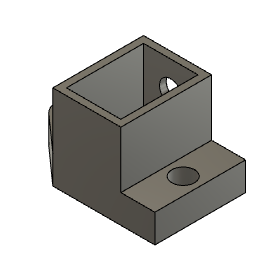
drawing_28 (Autodesk Fusion 360 design; units mm, degrees)
Autodesk Fusion 360 part; units mm, degrees
sketch "Sketch1" plane through (0, 0, 0) normal (0, 1, 0) x (1, 0, 0)
  line L0 (-15, -40) -> (60, -40)
  line L1 (60, -40) -> (60, 40)
  line L2 (60, 40) -> (-15, 40)
  line L3 (-60, -40) -> (60, 40) construction
  line L4 (60, -40) -> (-60, 40) construction
  line L5 (-60, 0) -> (-45, 0) construction
  line L6 (-45, 0) -> (-45, 13.3333) construction
  line L7 (-15, -40) -> (-15, 40)
  line L8 (-47.3875, 11.2111) -> (-15, 40)
  line L9 (-47.3875, -11.2111) -> (-15, -40)
  arc A0 (-47.3875, 11.2111) -> (-47.3875, -11.2111) centre (-37.422, 0) ccw
  circle A1 centre (-37.422, 0) radius 10
  dimension "d1" = 120
  dimension "d2" = 80
  dimension "d3" = 15
  dimension "d4" = 20
  constraint horizontal L0
  constraint perpendicular L0 L1
  constraint parallel L0 L2
  constraint coincident L3 origin
  constraint coincident L4 origin
  constraint perpendicular L2 L6
  constraint coincident L8 L6.end
  constraint coincident L5.start L8
  constraint coincident L5.start L9
  constraint tangent L8 A0
  constraint tangent L9 A0
  constraint concentric A0 A1
  measures "d1" distance of L1.end L4.end
  measures "d2" distance of L0.end L1.end
  measures "d3" radius of A0
  measures "d4" diameter of A1
extrude "Extrude1" add sketch "Sketch1" along normal blind 25
extrude "Extrude2" add 1 faces at (60, 8.3333, 13.3333) along direction (1, 0, 0) blind 15
sketch "Sketch3" plane through (0, 25, 0) normal (0, 1, 0) x (-1, 0, 0)
  circle A0 centre (37.422, 0) radius 10
  arc A1 (47.3875, -11.2111) -> (47.3875, 11.2111) centre (37.422, 0) ccw
  line L0 (47.3875, 11.2111) -> (15, 40)
  line L1 (15, 40) -> (-75, 40)
  line L2 (-75, 40) -> (-75, -40)
  line L3 (-75, -40) -> (15, -40)
  line L4 (15, -40) -> (47.3875, -11.2111)
  line L5 (-75, 0) -> (-60, 0) construction
  circle A2 centre (-60, 0) radius 10
  dimension "d10" = 15
  dimension "d11" = 20
  constraint midpoint L2 L5.start
  constraint perpendicular L2 L5
  constraint coincident L5.end A2.centre
  measures "d10" distance of L5.start L5.end
  measures "d11" diameter of A2
extrude "Extrude3" cut sketch "Sketch3" against normal blind 55 contours A2
sketch "Sketch4" plane through (0, 25, 0) normal (0, 1, 0) x (-1, 0, 0)
  circle A0 centre (-60, 0) radius 10
  circle A1 centre (37.422, 0) radius 10
  arc A2 (47.3875, -11.2111) -> (47.3875, 11.2111) centre (37.422, 0) ccw
  line L0 (47.3875, 11.2111) -> (15, 40)
  line L1 (15, 40) -> (-75, 40)
  line L2 (-75, 40) -> (-75, -40)
  line L3 (-75, -40) -> (15, -40)
  line L4 (15, -40) -> (47.3875, -11.2111)
  line L5 (15, 40) -> (-45, 40)
  line L6 (-45, 40) -> (-45, -40)
  line L7 (-45, -40) -> (15, -40)
  line L8 (15, -40) -> (15, 40)
  line L9 (15, 40) -> (-45, -40) construction
  line L10 (-45, 40) -> (15, -40) construction
  point P0 (-15, 0)
  constraint horizontal L5
  constraint perpendicular L5 L6
  constraint parallel L5 L7
  constraint parallel L6 L8
  constraint coincident L0.end L1.start
  constraint coincident L9 P0
  constraint coincident L10 P0
extrude "Extrude4" add sketch "Sketch4" along normal blind 50 contours L1 L3 L5 L6 L7 L8
shell "Shell1" thickness 6 removed faces 1 at (5, 75, -13.3333)
sketch "Sketch5" plane through (0, 6, 0) normal (0, 1, 0) x (-1, 0, 0)
  line L0 (33.514, 15.5154) -> (12.7188, 34)
  line L1 (12.7188, 34) -> (-69, 34)
  line L2 (-69, 34) -> (-69, 13.2288)
  arc A0 (-69, -13.2288) -> (-69, 13.2288) centre (-60, 0) ccw
  line L3 (-69, -13.2288) -> (-69, -34)
  line L4 (-69, -34) -> (12.7188, -34)
  line L5 (12.7188, -34) -> (33.514, -15.5154)
  arc A1 (33.514, 15.5154) -> (33.514, -15.5154) centre (37.422, 0) ccw
  line L6 (-15, -40) -> (-15, -16) construction
  line L7 (-2.5, -3.5) -> (-27.5, -3.5)
  line L8 (-27.5, -3.5) -> (-27.5, -28.5)
  line L9 (-27.5, -28.5) -> (-2.5, -28.5)
  line L10 (-2.5, -28.5) -> (-2.5, -3.5)
  line L11 (-2.5, -3.5) -> (-27.5, -28.5) construction
  line L12 (-27.5, -3.5) -> (-2.5, -28.5) construction
  point P0 (-15, -16)
  dimension "d17" = 24
  dimension "d18" = 25
  dimension "d19" = 25
  constraint perpendicular L4 L6
  constraint horizontal L7
  constraint perpendicular L7 L8
  constraint parallel L7 L9
  constraint parallel L8 L10
  constraint coincident L11 P0
  constraint coincident L12 P0
  constraint coincident P0 L6.end
  measures "d17" distance of L6.start P0
  measures "d18" distance of L8.end L9.end
  measures "d19" distance of L7.end L8.end
extrude "Extrude5" cut sketch "Sketch5" against normal blind 200 contours L7 L8 L9 L10
sketch "Sketch6" plane through (0, 6, 0) normal (0, 1, 0) x (-1, 0, 0)
  line L0 (-27.5, -3.5) -> (-2.5, -3.5)
  line L1 (-2.5, -3.5) -> (-2.5, -28.5)
  line L2 (-2.5, -28.5) -> (-27.5, -28.5)
  line L3 (-27.5, -28.5) -> (-27.5, -3.5)
  line L4 (33.514, 15.5154) -> (12.7188, 34)
  line L5 (12.7188, 34) -> (-69, 34)
  line L6 (-69, 34) -> (-69, 13.2288)
  arc A0 (-69, -13.2288) -> (-69, 13.2288) centre (-60, 0) ccw
  line L7 (-69, -13.2288) -> (-69, -34)
  line L8 (-69, -34) -> (12.7188, -34)
  line L9 (12.7188, -34) -> (33.514, -15.5154)
  arc A1 (33.514, 15.5154) -> (33.514, -15.5154) centre (37.422, 0) ccw
  line L10 (-60, 0) -> (-15, 0) construction
  line L11 (-15, 0) -> (-15, 20) construction
  line L12 (-15, 20) -> (-15, 34) construction
  line L13 (-15, 34) -> (-15, 14) construction
  circle A2 centre (-15, 14) radius 9
  dimension "d22" = 20
  dimension "d23" = 18
  constraint coincident A0.centre L10.start
  constraint parallel L5 L10
  constraint perpendicular L5 L11
  constraint coincident L5 L12.end
  constraint perpendicular L5 L12
  constraint perpendicular L5 L13
  constraint coincident L13.end A2.centre
  measures "d22" distance of L12.end L13.end
  measures "d23" diameter of A2
extrude "Extrude6" cut sketch "Sketch6" against normal blind 200 contours A2
sketch "Sketch7" plane through (0, 0, -40) normal (0, 0, -1) x (-1, 0, 0)
  line L0 (-75, 0) -> (15, 0)
  line L1 (15, 0) -> (15, 25)
  line L2 (15, 25) -> (15, 75)
  line L3 (15, 75) -> (-45, 75)
  line L4 (-45, 75) -> (-45, 25)
  line L5 (-45, 25) -> (-75, 25)
  line L6 (-75, 25) -> (-75, 0)
  line L7 (15, 0) -> (-45, 0) construction
  line L8 (-15, 0) -> (-15, 50) construction
  circle A0 centre (-15, 50) radius 10
  dimension "d26" = 50
  dimension "d27" = 20
  constraint coincident L0.end L1.start
  constraint coincident L0 L7.end
  constraint midpoint L7 L8.start
  constraint perpendicular L7 L8
  constraint coincident L8.end A0.centre
  measures "d26" distance of L8.start L8.end
  measures "d27" diameter of A0
extrude "Extrude7" cut sketch "Sketch7" against normal blind 20 contours A0
